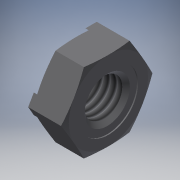
# Autodesk Inventor part: WLD-NUT DIN929 M8
Saved by Autodesk Inventor 2019.2 (Build 232265000, 265)
## iProperties
Category: PARTsolutions
Company: BOSSARD
Created: 2015-11-09
Part Number: WLD-NUT DIN929 M8
Catalog Web Link: www.cadenas.de
Description: Weld nut DIN929 M8
Vendor: BOSSARD
Document SubType Name: Modeling
Designer: psAdmin
Manufacturer: BOSSARD
Mass: 0.782802 g
Surface Area: 6.99141 cm^2
Volume: 0.782802 cm^3
Density: 1 g/cm^3
Material: Generic
Appearance: PSOLRGB-239-239-239
PSOL_IDENT_0: {$CADENAS_DATA\23d-libs\bossard\11\11_30\11_30_30\bn_31_10766\bn_10766.prj},257 {M=Nenngewinde},{VTY
PSOL_IDENT_1: P=3D},{NB=BN 10766 1716581 hexagon weld nut M8},{LINA=BN 10766 1716581 hexagon weld nut M8},{NN=BN 1
PSOL_IDENT_2: 0766},{DATE=07.05.2015 13:57:20},{GEOMDATE=28.01.2013 11:46:30},{VERSION=v1},{LINEID=60},{LINESUBID=
PSOL_IDENT_3: -1},{WBVAR=DIN962THREAD,DIN962OPT2}  {NB=BN 10766 1716581 hexagon weld nut M8},{LINA=BN 10766 171658
PSOL_IDENT_4: 1 hexagon weld nut M8},{KT=DUMMY},{NENN=M8},{CNSORDERNO=1716581},{BNARTNR=1716581},{BNNORM1=DIN 929}
PSOL_IDENT_5: ,{BNMAT=INOX A4},{CNSMAT=INOX A4},{BNSURFACE=},{GEW=M8},{D=8.000},{D1=6.647},{P=1.250},{DIN962THREAD=
PSOL_IDENT_6: },{DIN962THREAD1='', 'Rechtsgewinde', ' LH', 'Linksgewinde'},{XLH=0},{DIN962OPT2=},{B=1.000},{D2=10.
PSOL_IDENT_7: 500},{D3=10.500},{D4=8.400},{E=15.380},{H1=0.900},{H2=0.500},{M=6.500},{S=14.000},{VER=DIN 13},{SKD2=
PSOL_IDENT_8: 2.000},{OPTIONS2L='',' - ','din_962_std.jpg','-SK','SK Drahtloch','din_962_s_4.jpg'},{DIN962FTHREAD=
PSOL_IDENT_9: 0}
NN: BN 10766
NT: Hex weld nuts (DIN 929), A4, stainless steel A4
NB: BN 10766 1716581 hexagon weld nut M8
NBSYN: BN 10766 $BNARTNR. hexagon weld nut $NENN.
LINA: BN 10766 1716581 hexagon weld nut M8
ROWDESC: M8
OFFICIAL_STANDARD_NUMBERS: DIN 929
BNARTNR: 1716581
BNNORM1: DIN 929
BNMAT: INOX A4
D: 8.000
D1: 6.647
P: 1.250
B: 1.000
D2: 10.500
D3: 10.500
D4: 8.400
E: 15.380
H1: 0.900
H2: 0.500
M: 6.500
S: 14.000
SUPPLIER: BOSSARD
ARTICLENO: BN 10766 1716581 hexagon weld nut M8
BOMINFO: BN 10766 1716581 hexagon weld nut M8
CREATOR: CADENAS GmbH
Title: BN 10766 1716581 hexagon weld nut M8
Author: Cadenas PARTsolutions
Comments: Hex weld nuts (DIN 929), A4, stainless steel A4
Autodesk Inventor part; units mm, degrees
sketch "Skizze_1" plane through (0, 0, 0) normal (0, 0, 1) x (1, 0, 0)
  line L0 (5.6, 0) -> (-0.9, 0)
  line L1 (-0.9, 0) -> (-0.9, 8.4)
  line L2 (-0.9, 8.4) -> (5.6, 8.4)
  line L3 (5.6, 8.4) -> (5.6, 0)
  line L4 (5.6, 0) -> (-0.9, 0)
  constraints: 10 end point
revolve "Revolution1" add sketch "Skizze_1" angle 360 about axis through (5.6, 0, 0) along (1, 0, 0)
sketch "Sketch_6" plane through (0, 0, 0) normal (0, 0, 1) x (1, 0, 0)
  line L0 (5.6, 0) -> (-0.9, 0)
  line L1 (-0.9, 8.4) -> (-0.9, 5.25)
  line L2 (-0.9, 5.25) -> (-0.4, 5.25)
  line L3 (-0.4, 5.25) -> (-0.4, 8.4)
  line L4 (-0.4, 8.4) -> (-0.9, 8.4)
  constraints: 10 end point
revolve "Revolution2" cut sketch "Sketch_6" angle 360 about axis through (5.6, 0, 0) along (1, 0, 0)
sketch "Skizze_4" plane through (0, 0, 0) normal (0, 0, 1) x (1, 0, 0)
  line L0 (5.4, 0) -> (-0.9, 0)
  line L1 (-0.9, 0) -> (-0.9, 4)
  line L2 (-0.9, 4) -> (-0.2235, 3.3235)
  line L3 (-0.2235, 3.3235) -> (4.7235, 3.3235)
  line L4 (4.7235, 3.3235) -> (5.4, 4)
  line L5 (5.4, 4) -> (5.6, 4)
  line L6 (5.6, 4) -> (5.6, 0)
  line L7 (5.6, 0) -> (-0.9, 0)
  constraints: 16 end point
revolve "Revolution3" cut sketch "Skizze_4" angle 360 about axis through (5.4, 0, 0) along (1, 0, 0)
thread "Thread1" size "M8x1.25" class "6H" standard "ISO Metric profile" full length
sketch "Sketch_1" plane through (0, 0, 0) normal (0, 0, 1) x (1, 0, 0)
  line L0 (0, 0) -> (-0.9, 0)
  line L1 (-0.9, 8.4) -> (-0.9, 5.25)
  line L2 (-0.9, 5.25) -> (0, 5.25)
  line L3 (0, 5.25) -> (0, 8.4)
  line L4 (0, 8.4) -> (-0.9, 8.4)
  constraints: 10 end point
revolve "Revolution4" cut sketch "Sketch_1" angle 360 about axis through (0, 0, 0) along (1, 0, 0)
sketch "Sketch_2" plane through (0, 0, 0) normal (0, 0, 1) x (1, 0, 0)
  line L0 (5.6, 0) -> (-0.9, 0)
  line L1 (-0.9, 14.69) -> (-0.9, 7)
  line L2 (-0.9, 7) -> (0, 7)
  line L3 (0, 7) -> (0.3751, 8.4)
  line L4 (0.3751, 8.4) -> (5.2249, 8.4)
  line L5 (5.2249, 8.4) -> (5.6, 7)
  line L6 (5.6, 7) -> (6.5, 7)
  line L7 (6.5, 7) -> (6.5, 14.69)
  line L8 (6.5, 14.69) -> (-0.9, 14.69)
  constraints: 18 end point
revolve "Revolution5" cut sketch "Sketch_2" angle 360 about axis through (5.6, 0, 0) along (1, 0, 0)
sketch "Sketch_3" plane through (0, 0, 0) normal (0, 0, 1) x (1, 0, 0)
  line L0 (5.6, 0) -> (5.4, 0)
  line L1 (5.4, 0) -> (5.4, 5.25)
  line L2 (5.4, 5.25) -> (5.6, 5.25)
  line L3 (5.6, 5.25) -> (5.6, 0)
  line L4 (5.6, 0) -> (5.4, 0)
  constraints: 10 end point
revolve "Revolution6" cut sketch "Sketch_3" angle 360 about axis through (5.6, 0, 0) along (1, 0, 0)
sketch "Skizze_3" plane through (-0.5, 0, 0) normal (1, 0, 0) x (0, 0, -1)
  line L0 (-1.7321, -7.0829) -> (0, -8.0829)
  line L1 (0, -8.0829) -> (1.7321, -7.0829)
  line L2 (1.7321, -7.0829) -> (-1.7321, -7.0829)
  constraints: 6 end point
sketch "Skizze_9" plane through (-0.5, 0, 0) normal (1, 0, 0) x (0, 0, -1)
  line L0 (-7, 2.0415) -> (-5.2679, 5.0415)
  line L1 (-5.2679, 5.0415) -> (-7, 4.0415)
  line L2 (-7, 4.0415) -> (-7, 2.0415)
  constraints: 6 end point
sketch "Skizze_10" plane through (-0.5, 0, 0) normal (1, 0, 0) x (0, 0, -1)
  line L0 (5.2679, 5.0415) -> (7, 2.0415)
  line L1 (7, 2.0415) -> (7, 4.0415)
  line L2 (7, 4.0415) -> (5.2679, 5.0415)
  constraints: 6 end point
extrude "Extrusion1" add sketch "Skizze_3" along normal blind 2.1667
extrude "Extrusion2" add sketch "Skizze_9" along normal blind 2.1667
extrude "Extrusion3" add sketch "Skizze_10" along normal blind 2.1667
sketch "Skizze_7" plane through (0, 0, 0) normal (1, 0, 0) x (0, 1, 0)
  line L0 (15.38, 15.38) -> (-15.38, 15.38)
  line L1 (-15.38, 15.38) -> (-15.38, -15.38)
  line L2 (-15.38, -15.38) -> (15.38, -15.38)
  line L3 (15.38, -15.38) -> (15.38, 15.38)
  line L4 (-4.0415, 7) -> (-8.0829, 0)
  line L5 (-8.0829, 0) -> (-4.0415, -7)
  line L6 (-4.0415, -7) -> (4.0415, -7)
  line L7 (4.0415, -7) -> (8.0829, 0)
  line L8 (8.0829, 0) -> (4.0415, 7)
  line L9 (4.0415, 7) -> (-4.0415, 7)
  constraints: 20 end point
extrude "Extrusion4" cut sketch "Skizze_7" along normal mid plane 13
ref_plane "IP1_XY" through (0, 0, 0) normal (1, 0, 0) x (0, 0, -1)
ref_plane "IP1_YZ" through (0, 0, 0) normal (0, 0, -1) x (0, 1, 0)
ref_plane "IP1_ZX" through (0, 0, 0) normal (0, 1, 0) x (1, 0, 0)
ref_plane "IP2_XY" through (5.6, 0, 0) normal (1, 0, 0) x (0, 0, -1)
ref_plane "IP2_YZ" through (5.6, 0, 0) normal (0, 0, -1) x (0, 1, 0)
ref_plane "IP2_ZX" through (5.6, 0, 0) normal (0, 1, 0) x (1, 0, 0)
body "Solid1"
